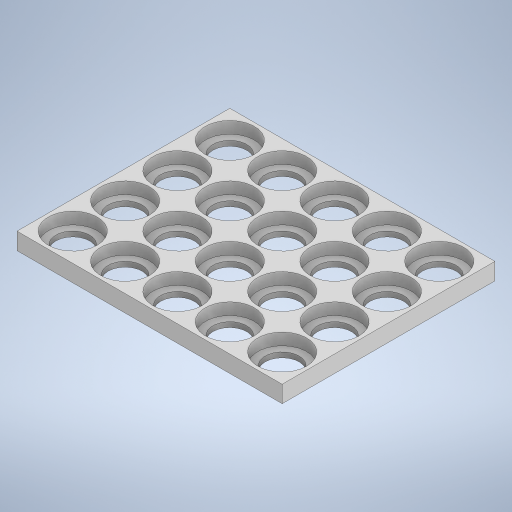
# Autodesk Inventor part: battery_pack_base
Saved by Autodesk Inventor 2023 (Build 270158000, 158)
## iProperties
Created: 2024-04-10
Part Number: battery_pack_base
Material: Genérico
Document SubType Name: Modeling
Designer: inigo
Density: 1 g/cm^3
Appearance: Valor por defecto
Author: inigo
Autodesk Inventor part; units mm, degrees
ref_plane "YZ Plane" through (0, 0, 0) normal (1, 0, 0) x (0, 1, 0)
ref_plane "XZ Plane" through (0, 0, 0) normal (0, 1, 0) x (-1, 0, 0)
ref_plane "XY Plane" through (0, 0, 0) normal (0, 0, 1) x (1, 0, 0)
sketch "Boceto1" plane through (0, 0, 0) normal (0, 1, 0) x (-1, 0, 0)
  line L0 (39.25, 31.5) -> (-39.25, 31.5)
  line L1 (-39.25, 31.5) -> (-39.25, -31.5)
  line L2 (-39.25, -31.5) -> (39.25, -31.5)
  line L3 (39.25, -31.5) -> (39.25, 31.5)
  line L4 (39.25, 31.5) -> (-39.25, -31.5) construction
  line L5 (-39.25, 31.5) -> (39.25, -31.5) construction
  point P0 (0, 0)
  dimension "d0" = 78.5
  dimension "d1" = 63
  constraints: 12 end point, 2 midpoint, 2 parallel, 1 horizontal, 1 perpendicular
  measures "d0" distance of L2.end L1.end
  measures "d1" distance of L1.end L0.end
extrude "Extrusión1" add sketch "Boceto1" along normal blind 5
sketch "Boceto2" plane through (0, 5, 0) normal (0, 1, 0) x (1, 0, 0)
  circle A0 centre (31, -23.25) radius 7.25
  line L0 (0, 0) -> (0, -1.7079)
  line L1 (-39.25, -31.5) -> (39.25, -31.5) projected
  line L2 (0, 0) -> (-6.7024, 0)
  line L3 (31, -30.5) -> (-1.6149, -30.5)
  line L4 (38.25, -23.25) -> (38.25, -18.8527)
  line L5 (39.25, -31.5) -> (39.25, 31.5) projected
  line L6 (31, -23.25) -> (31, -17.7026)
  line L7 (31, -16) -> (21.1009, -16)
  line L8 (31, -0.5) -> (21.1009, -0.5)
  circle A1 centre (31, -7.75) radius 7.25
  line L9 (31, -15) -> (-1.6149, -15)
  line L10 (31, 15) -> (21.1009, 15)
  circle A2 centre (31, 7.75) radius 7.25
  line L11 (31, 0.5) -> (-1.6149, 0.5)
  line L12 (31, 30.5) -> (21.1009, 30.5)
  circle A3 centre (31, 23.25) radius 7.25
  line L13 (31, 16) -> (-1.6149, 16)
  line L14 (39.25, 31.5) -> (-39.25, 31.5) projected
  circle A4 centre (15.5, -23.25) radius 7.25
  circle A5 centre (15.5, -7.75) radius 7.25
  circle A6 centre (15.5, 7.75) radius 7.25
  circle A7 centre (15.5, 23.25) radius 7.25
  circle A8 centre (0, -23.25) radius 7.25
  circle A9 centre (0, -7.75) radius 7.25
  circle A10 centre (0, 7.75) radius 7.25
  circle A11 centre (0, 23.25) radius 7.25
  circle A12 centre (-15.5, -23.25) radius 7.25
  circle A13 centre (-15.5, -7.75) radius 7.25
  circle A14 centre (-15.5, 7.75) radius 7.25
  circle A15 centre (-15.5, 23.25) radius 7.25
  circle A16 centre (-31, -23.25) radius 7.25
  circle A17 centre (-31, -7.75) radius 7.25
  circle A18 centre (-31, 7.75) radius 7.25
  circle A19 centre (-31, 23.25) radius 7.25
  line L15 (22.75, -23.25) -> (22.75, -18.6411)
  line L16 (23.75, -23.25) -> (23.75, -18.1365)
  line L17 (-38.25, -23.25) -> (-38.25, -18.441)
  line L18 (-39.25, 31.5) -> (-39.25, -31.5) projected
  point P0 (-1.5837, 0)
  point P1 (38.25, -7.75)
  point P2 (38.25, 7.75)
  point P3 (38.25, 23.25)
  point P4 (15.5, -30.5)
  point P5 (15.5, -16)
  point P6 (15.5, -15)
  point P7 (22.75, -7.75)
  point P8 (15.5, -0.5)
  point P9 (15.5, 0.5)
  point P10 (22.75, 7.75)
  point P11 (15.5, 15)
  point P12 (15.5, 16)
  point P13 (22.75, 23.25)
  point P14 (15.5, 30.5)
  point P15 (0, -30.5)
  point P16 (7.25, -23.25)
  point P17 (0, -16)
  point P18 (0, -15)
  point P19 (7.25, -7.75)
  point P20 (0, -0.5)
  point P21 (0, 0.5)
  point P22 (7.25, 7.75)
  point P23 (0, 15)
  point P24 (0, 16)
  point P25 (7.25, 23.25)
  point P26 (0, 30.5)
  point P27 (-15.5, -30.5)
  point P28 (-8.25, -23.25)
  point P29 (-15.5, -16)
  point P30 (-15.5, -15)
  point P31 (-8.25, -7.75)
  point P32 (-15.5, -0.5)
  point P33 (-15.5, 0.5)
  point P34 (-8.25, 7.75)
  point P35 (-15.5, 15)
  point P36 (-15.5, 16)
  point P37 (-8.25, 23.25)
  point P38 (-15.5, 30.5)
  point P39 (-31, -30.5)
  point P40 (-23.75, -23.25)
  point P41 (-31, -16)
  point P42 (-31, -15)
  point P43 (-23.75, -7.75)
  point P44 (-31, -0.5)
  point P45 (-31, 0.5)
  point P46 (-23.75, 7.75)
  point P47 (-31, 15)
  point P48 (-31, 16)
  point P49 (-23.75, 23.25)
  point P50 (-31, 30.5)
  dimension "d4" = 14.5
  dimension "d6" = 23.25
  dimension "d13" = 7.25
  dimension "d14" = 1
  dimension "d15" = 7.25
  dimension "d16" = 1
  dimension "d19" = 15.5
  dimension "d24" = 1
  dimension "d25" = 1
  dimension "d28" = 15.5
  dimension "d33" = 1
  dimension "d34" = 1
  constraints: 62 point on circle, 30 end point, 20 centre point, 7 vertical, 5 tangent, 3 horizontal, 107 other
  measures "d4" diameter of A0
  measures "d6" vertical distance of point (-1.584, 0) L6.start
  measures "d13" distance from line of L3 L6.start
  measures "d14" distance between parallel lines of L1 L3
  measures "d15" distance from line of L6.start L4
  measures "d16" distance between parallel lines of L5 L4
  measures "d19" distance of L7.start L8.start
  measures "d24" distance between parallel lines of L7 L9
  measures "d25" distance between parallel lines of L14 L12
  measures "d28" distance of L6.start A4.centre
  measures "d33" distance between parallel lines of L16 L15
  measures "d34" distance between parallel lines of L18 L17
extrude "Extrusión2" cut sketch "Boceto2" against normal blind 3.5 contours A0 | A8 | A4 | A1 | A9 | A5 | A2 | A10 | A6 | A3 | A11 | A7 | A12 | A13 | A14 | A15 | A16 | A17 | A18 | A19
sketch "Boceto3" plane through (31, 1.5, 23.25) normal (0, 1, 0) x (1, 0, 0)
  circle A0 centre (0, 0) radius 5
  line L0 (0, 0) -> (0, 5.1334)
  circle A1 centre (0, 15.5) radius 5
  circle A2 centre (0, 31) radius 5
  circle A3 centre (0, 46.5) radius 5
  circle A4 centre (0, 15.5) radius 7.25
  line L1 (0, 0) -> (-4.4758, 0)
  circle A5 centre (-15.5, 46.5) radius 5
  circle A6 centre (-15.5, 31) radius 5
  circle A7 centre (-15.5, 15.5) radius 5
  circle A8 centre (-15.5, 0) radius 5
  circle A9 centre (-31, 46.5) radius 5
  circle A10 centre (-31, 31) radius 5
  circle A11 centre (-31, 15.5) radius 5
  circle A12 centre (-31, 0) radius 5
  circle A13 centre (-46.5, 46.5) radius 5
  circle A14 centre (-46.5, 31) radius 5
  circle A15 centre (-46.5, 15.5) radius 5
  circle A16 centre (-46.5, 0) radius 5
  circle A17 centre (-62, 46.5) radius 5
  circle A18 centre (-62, 31) radius 5
  circle A19 centre (-62, 15.5) radius 5
  circle A20 centre (-62, 0) radius 5
  circle A21 centre (-15.5, 0) radius 7.25
  circle A22 centre (0, 0) radius 7.25 projected
  point P0 (-31, 23.25)
  dimension "d10" = 10
  dimension "d37" = 15.5
  dimension "d44" = 15.5
  dimension "d49" = 2.25
  constraints: 22 centre point, 4 end point, 2 coincident, 2 horizontal, 2 vertical, 38 other
  measures "d10" diameter of A0
  measures "d37" distance of L0.start A1.centre
  measures "d44" distance of A3.centre A5.centre
  measures "d49" radial gap between concentric circles of A22 A0
extrude "Extrusión3" cut sketch "Boceto3" against normal blind 4 contours A0 | A1 | A2 | A3 | A5 | A6 | A7 | A8 | A9 | A10 | A11 | A12 | A13 | A14 | A15 | A16 | A17 | A18 | A19 | A20
